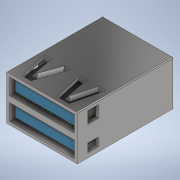
# Autodesk Inventor part: Port 2
Saved by Autodesk Inventor 2020 (Build 240168000, 168)
## iProperties
Created: 2022-11-24
Part Number: Port 2
Material: Generic
Document SubType Name: Modeling
Designer: DELL
Density: 1 g/cm^3
Appearance: Steel - Polished
Author: DELL
Autodesk Inventor part; units mm, degrees
ref_plane "YZ Plane" through (0, 0, 0) normal (1, 0, 0) x (0, 1, 0)
ref_plane "XZ Plane" through (0, 0, 0) normal (0, 1, 0) x (-1, 0, 0)
ref_plane "XY Plane" through (0, 0, 0) normal (0, 0, 1) x (1, 0, 0)
sketch "Sketch1" plane through (0, 0, 0) normal (0, 1, 0) x (-1, 0, 0)
  line L0 (0, 0) -> (0, 32.4)
  line L1 (0, 32.4) -> (-23.897, 32.4)
  line L2 (-23.897, 32.4) -> (-23.897, 0)
  line L3 (-23.897, 0) -> (0, 0)
  dimension "d1" = 32.4
  dimension "d2" = 23.897
  constraints: 8 end point, 3 perpendicular, 1 vertical
  measures "d1" distance of L0.start L0.end
  measures "d2" distance of L0.end L1.end
extrude "Extrusion1" add sketch "Sketch1" along normal blind 15
sketch "Sketch2" plane through (0, 0, 32.4) normal (0, 0, 1) x (1, 0, 0)
  line L0 (23.897, 0) -> (23.897, 15) projected
  line L1 (23.897, 0) -> (0, 0) projected
  line L2 (1, 14) -> (1, 1)
  line L3 (22.897, 14) -> (22.897, 1)
  line L4 (22.897, 14) -> (1, 14)
  line L5 (22.897, 1) -> (1, 1)
  line L6 (1, 14) -> (1, 8.5)
  line L7 (1, 8.5) -> (22.897, 8.5)
  line L8 (1, 1) -> (1, 6.5)
  line L9 (1, 6.5) -> (22.897, 6.5)
  line L10 (1, 14) -> (2, 14)
  line L11 (22.897, 14) -> (21.897, 14)
  line L12 (1, 14) -> (1, 13)
  line L13 (1, 8.5) -> (1, 9.5)
  line L14 (2, 13) -> (2, 9.5)
  line L15 (2, 9.5) -> (21.897, 9.5)
  line L16 (21.897, 9.5) -> (21.897, 13)
  line L17 (21.897, 13) -> (2, 13)
  line L18 (1, 6.5) -> (2, 6.5)
  line L19 (22.897, 6.5) -> (21.897, 6.5)
  line L20 (1, 6.5) -> (1, 5.5)
  line L21 (1, 1) -> (1, 2)
  line L22 (2, 5.5) -> (21.897, 5.5)
  line L23 (21.897, 5.5) -> (21.897, 2)
  line L24 (21.897, 2) -> (2, 2)
  line L25 (2, 2) -> (2, 5.5)
  line L26 (2.5159, 9.5) -> (2.8749, 9.5)
  line L27 (2.8749, 9.5) -> (2.8749, 9.2899)
  line L28 (2.8749, 9.2899) -> (2.5159, 9.2899)
  line L29 (2.5159, 9.2899) -> (2.5159, 9.5)
  line L30 (3.5159, 9.5) -> (3.8749, 9.5)
  line L31 (3.5159, 9.2899) -> (3.5159, 9.5)
  line L32 (3.8749, 9.5) -> (3.8749, 9.2899)
  line L33 (3.8749, 9.2899) -> (3.5159, 9.2899)
  line L34 (4.5159, 9.5) -> (4.8749, 9.5)
  line L35 (4.5159, 9.2899) -> (4.5159, 9.5)
  line L36 (4.8749, 9.5) -> (4.8749, 9.2899)
  line L37 (4.8749, 9.2899) -> (4.5159, 9.2899)
  line L38 (5.5159, 9.5) -> (5.8749, 9.5)
  line L39 (5.5159, 9.2899) -> (5.5159, 9.5)
  line L40 (5.8749, 9.5) -> (5.8749, 9.2899)
  line L41 (5.8749, 9.2899) -> (5.5159, 9.2899)
  line L42 (6.5159, 9.5) -> (6.8749, 9.5)
  line L43 (6.5159, 9.2899) -> (6.5159, 9.5)
  line L44 (6.8749, 9.5) -> (6.8749, 9.2899)
  line L45 (6.8749, 9.2899) -> (6.5159, 9.2899)
  line L46 (7.5159, 9.5) -> (7.8749, 9.5)
  line L47 (7.5159, 9.2899) -> (7.5159, 9.5)
  line L48 (7.8749, 9.5) -> (7.8749, 9.2899)
  line L49 (7.8749, 9.2899) -> (7.5159, 9.2899)
  line L50 (8.5159, 9.5) -> (8.8749, 9.5)
  line L51 (8.5159, 9.2899) -> (8.5159, 9.5)
  line L52 (8.8749, 9.5) -> (8.8749, 9.2899)
  line L53 (8.8749, 9.2899) -> (8.5159, 9.2899)
  line L54 (9.5159, 9.5) -> (9.8749, 9.5)
  line L55 (9.5159, 9.2899) -> (9.5159, 9.5)
  line L56 (9.8749, 9.5) -> (9.8749, 9.2899)
  line L57 (9.8749, 9.2899) -> (9.5159, 9.2899)
  line L58 (10.5159, 9.5) -> (10.8749, 9.5)
  line L59 (10.5159, 9.2899) -> (10.5159, 9.5)
  line L60 (10.8749, 9.5) -> (10.8749, 9.2899)
  line L61 (10.8749, 9.2899) -> (10.5159, 9.2899)
  line L62 (11.5159, 9.5) -> (11.8749, 9.5)
  line L63 (11.5159, 9.2899) -> (11.5159, 9.5)
  line L64 (11.8749, 9.5) -> (11.8749, 9.2899)
  line L65 (11.8749, 9.2899) -> (11.5159, 9.2899)
  line L66 (12.5159, 9.5) -> (12.8749, 9.5)
  line L67 (12.5159, 9.2899) -> (12.5159, 9.5)
  line L68 (12.8749, 9.5) -> (12.8749, 9.2899)
  line L69 (12.8749, 9.2899) -> (12.5159, 9.2899)
  line L70 (13.5159, 9.5) -> (13.8749, 9.5)
  line L71 (13.5159, 9.2899) -> (13.5159, 9.5)
  line L72 (13.8749, 9.5) -> (13.8749, 9.2899)
  line L73 (13.8749, 9.2899) -> (13.5159, 9.2899)
  line L74 (14.5159, 9.5) -> (14.8749, 9.5)
  line L75 (14.5159, 9.2899) -> (14.5159, 9.5)
  line L76 (14.8749, 9.5) -> (14.8749, 9.2899)
  line L77 (14.8749, 9.2899) -> (14.5159, 9.2899)
  line L78 (15.5159, 9.5) -> (15.8749, 9.5)
  line L79 (15.5159, 9.2899) -> (15.5159, 9.5)
  line L80 (15.8749, 9.5) -> (15.8749, 9.2899)
  line L81 (15.8749, 9.2899) -> (15.5159, 9.2899)
  line L82 (16.5159, 9.5) -> (16.8749, 9.5)
  line L83 (16.5159, 9.2899) -> (16.5159, 9.5)
  line L84 (16.8749, 9.5) -> (16.8749, 9.2899)
  line L85 (16.8749, 9.2899) -> (16.5159, 9.2899)
  line L86 (17.5159, 9.5) -> (17.8749, 9.5)
  line L87 (17.5159, 9.2899) -> (17.5159, 9.5)
  line L88 (17.8749, 9.5) -> (17.8749, 9.2899)
  line L89 (17.8749, 9.2899) -> (17.5159, 9.2899)
  line L90 (18.5159, 9.5) -> (18.8749, 9.5)
  line L91 (18.5159, 9.2899) -> (18.5159, 9.5)
  line L92 (18.8749, 9.5) -> (18.8749, 9.2899)
  line L93 (18.8749, 9.2899) -> (18.5159, 9.2899)
  line L94 (19.5159, 9.5) -> (19.8749, 9.5)
  line L95 (19.5159, 9.2899) -> (19.5159, 9.5)
  line L96 (19.8749, 9.5) -> (19.8749, 9.2899)
  line L97 (19.8749, 9.2899) -> (19.5159, 9.2899)
  line L98 (20.5159, 9.5) -> (20.8749, 9.5)
  line L99 (20.5159, 9.2899) -> (20.5159, 9.5)
  line L100 (20.8749, 9.5) -> (20.8749, 9.2899)
  line L101 (20.8749, 9.2899) -> (20.5159, 9.2899)
  line L102 (21.5159, 9.5) -> (21.8749, 9.5)
  line L103 (21.5159, 9.2899) -> (21.5159, 9.5)
  line L104 (21.8749, 9.5) -> (21.8749, 9.2899)
  line L105 (21.8749, 9.2899) -> (21.5159, 9.2899)
  line L106 (2, 2) -> (2.516, 2)
  line L107 (2.516, 2) -> (2.7683, 2)
  line L108 (2.7683, 2) -> (2.7683, 1.8627)
  line L109 (2.7683, 1.8627) -> (2.516, 1.8627)
  line L110 (2.516, 1.8627) -> (2.516, 2)
  line L111 (22.797, 2) -> (2.9, 2)
  line L112 (3.6683, 2) -> (3.6683, 1.8627)
  line L113 (3.416, 2) -> (3.6683, 2)
  line L114 (3.416, 1.8627) -> (3.416, 2)
  line L115 (3.6683, 1.8627) -> (3.416, 1.8627)
  line L116 (23.697, 2) -> (3.8, 2)
  line L117 (4.5683, 2) -> (4.5683, 1.8627)
  line L118 (4.316, 2) -> (4.5683, 2)
  line L119 (4.316, 1.8627) -> (4.316, 2)
  line L120 (4.5683, 1.8627) -> (4.316, 1.8627)
  line L121 (24.597, 2) -> (4.7, 2)
  line L122 (5.4683, 2) -> (5.4683, 1.8627)
  line L123 (5.216, 2) -> (5.4683, 2)
  line L124 (5.216, 1.8627) -> (5.216, 2)
  line L125 (5.4683, 1.8627) -> (5.216, 1.8627)
  line L126 (25.497, 2) -> (5.6, 2)
  line L127 (6.3683, 2) -> (6.3683, 1.8627)
  line L128 (6.116, 2) -> (6.3683, 2)
  line L129 (6.116, 1.8627) -> (6.116, 2)
  line L130 (6.3683, 1.8627) -> (6.116, 1.8627)
  line L131 (26.397, 2) -> (6.5, 2)
  line L132 (7.2683, 2) -> (7.2683, 1.8627)
  line L133 (7.016, 2) -> (7.2683, 2)
  line L134 (7.016, 1.8627) -> (7.016, 2)
  line L135 (7.2683, 1.8627) -> (7.016, 1.8627)
  line L136 (27.297, 2) -> (7.4, 2)
  line L137 (8.1683, 2) -> (8.1683, 1.8627)
  line L138 (7.916, 2) -> (8.1683, 2)
  line L139 (7.916, 1.8627) -> (7.916, 2)
  line L140 (8.1683, 1.8627) -> (7.916, 1.8627)
  line L141 (28.197, 2) -> (8.3, 2)
  line L142 (9.0683, 2) -> (9.0683, 1.8627)
  line L143 (8.816, 2) -> (9.0683, 2)
  line L144 (8.816, 1.8627) -> (8.816, 2)
  line L145 (9.0683, 1.8627) -> (8.816, 1.8627)
  line L146 (29.097, 2) -> (9.2, 2)
  line L147 (9.9683, 2) -> (9.9683, 1.8627)
  line L148 (9.716, 2) -> (9.9683, 2)
  line L149 (9.716, 1.8627) -> (9.716, 2)
  line L150 (9.9683, 1.8627) -> (9.716, 1.8627)
  line L151 (29.997, 2) -> (10.1, 2)
  line L152 (10.8683, 2) -> (10.8683, 1.8627)
  line L153 (10.616, 2) -> (10.8683, 2)
  line L154 (10.616, 1.8627) -> (10.616, 2)
  line L155 (10.8683, 1.8627) -> (10.616, 1.8627)
  line L156 (30.897, 2) -> (11, 2)
  line L157 (11.7683, 2) -> (11.7683, 1.8627)
  line L158 (11.516, 2) -> (11.7683, 2)
  line L159 (11.516, 1.8627) -> (11.516, 2)
  line L160 (11.7683, 1.8627) -> (11.516, 1.8627)
  line L161 (31.797, 2) -> (11.9, 2)
  line L162 (12.6683, 2) -> (12.6683, 1.8627)
  line L163 (12.416, 2) -> (12.6683, 2)
  line L164 (12.416, 1.8627) -> (12.416, 2)
  line L165 (12.6683, 1.8627) -> (12.416, 1.8627)
  line L166 (32.697, 2) -> (12.8, 2)
  line L167 (13.5683, 2) -> (13.5683, 1.8627)
  line L168 (13.316, 2) -> (13.5683, 2)
  line L169 (13.316, 1.8627) -> (13.316, 2)
  line L170 (13.5683, 1.8627) -> (13.316, 1.8627)
  line L171 (33.597, 2) -> (13.7, 2)
  line L172 (14.4683, 2) -> (14.4683, 1.8627)
  line L173 (14.216, 2) -> (14.4683, 2)
  line L174 (14.216, 1.8627) -> (14.216, 2)
  line L175 (14.4683, 1.8627) -> (14.216, 1.8627)
  line L176 (34.497, 2) -> (14.6, 2)
  line L177 (15.3683, 2) -> (15.3683, 1.8627)
  line L178 (15.116, 2) -> (15.3683, 2)
  line L179 (15.116, 1.8627) -> (15.116, 2)
  line L180 (15.3683, 1.8627) -> (15.116, 1.8627)
  line L181 (35.397, 2) -> (15.5, 2)
  line L182 (16.2683, 2) -> (16.2683, 1.8627)
  line L183 (16.016, 2) -> (16.2683, 2)
  line L184 (16.016, 1.8627) -> (16.016, 2)
  line L185 (16.2683, 1.8627) -> (16.016, 1.8627)
  line L186 (36.297, 2) -> (16.4, 2)
  line L187 (17.1683, 2) -> (17.1683, 1.8627)
  line L188 (16.916, 2) -> (17.1683, 2)
  line L189 (16.916, 1.8627) -> (16.916, 2)
  line L190 (17.1683, 1.8627) -> (16.916, 1.8627)
  line L191 (37.197, 2) -> (17.3, 2)
  line L192 (18.0683, 2) -> (18.0683, 1.8627)
  line L193 (17.816, 2) -> (18.0683, 2)
  line L194 (17.816, 1.8627) -> (17.816, 2)
  line L195 (18.0683, 1.8627) -> (17.816, 1.8627)
  line L196 (38.097, 2) -> (18.2, 2)
  line L197 (18.9683, 2) -> (18.9683, 1.8627)
  line L198 (18.716, 2) -> (18.9683, 2)
  line L199 (18.716, 1.8627) -> (18.716, 2)
  line L200 (18.9683, 1.8627) -> (18.716, 1.8627)
  line L201 (38.997, 2) -> (19.1, 2)
  line L202 (19.8683, 2) -> (19.8683, 1.8627)
  line L203 (19.616, 2) -> (19.8683, 2)
  line L204 (19.616, 1.8627) -> (19.616, 2)
  line L205 (19.8683, 1.8627) -> (19.616, 1.8627)
  line L206 (39.897, 2) -> (20, 2)
  line L207 (20.7683, 2) -> (20.7683, 1.8627)
  line L208 (20.516, 2) -> (20.7683, 2)
  line L209 (20.516, 1.8627) -> (20.516, 2)
  line L210 (20.7683, 1.8627) -> (20.516, 1.8627)
  line L211 (40.797, 2) -> (20.9, 2)
  line L212 (21.6683, 2) -> (21.6683, 1.8627)
  line L213 (21.416, 2) -> (21.6683, 2)
  line L214 (21.416, 1.8627) -> (21.416, 2)
  line L215 (21.6683, 1.8627) -> (21.416, 1.8627)
  point P0 (0, 15)
  dimension "d9" = 5.5
  dimension "d10" = 5.5
  dimension "d11" = 1
  dimension "d13" = 1
  dimension "d14" = 1
  dimension "d15" = 1
  dimension "d17" = 1
  dimension "d18" = 1
  dimension "d21" = 1
  dimension "d26" = 0.516
  dimension "d29" = 0.9
  constraints: 424 end point, 202 horizontal alignment, 100 collinear, 84 parallel, 33 point on line, 4 perpendicular, 3 horizontal, 1 vertical, 8 other
  measures "d9" distance of L2.start L6.end
  measures "d10" distance of L2.end L8.end
  measures "d11" distance of L2.start L10.end
  measures "d13" distance of L2.start L12.end
  measures "d14" distance of L6.end L13.end
  measures "d15" distance of L8.end L18.end
  measures "d17" distance of L8.end L20.end
  measures "d18" distance of L2.end L21.end
  measures "d21" distance of L26.start L30.start
  measures "d26" distance of L25.start L106.end
  measures "d29" distance of L23.end L111.start
extrude "Extrusion2" cut sketch "Sketch2" against normal blind 30 contours L4 L3 L7 L2
extrude "Extrusion3" cut sketch "Sketch2" against normal blind 30 contours L9 L3 L5 L2
extrude "Extrusion4" cut sketch "Sketch2" along normal blind 3 contours L17 L16 L15 L14
extrude "Extrusion5" cut sketch "Sketch2" against normal blind 1 contours L24 L25 L22 L23 | L17 L16 L15 L14
extrude "Extrusion6" cut sketch "Sketch2" against normal blind 1.2 contours L15 L27 L28 L29 | L15 L32 L33 L31 | L15 L36 L37 L35 | L15 L40 L41 L39 | L15 L44 L45 L43 | L15 L48 L49 L47 | L15 L52 L53 L51 | L15 L56 L57 L55 | L15 L60 L61 L59 | L72 L73 L71 L15 | L15 L64 L65 L63 | L68 L69 L67 L15
extrude "Extrusion7" cut sketch "Sketch2" against normal blind 1.2 contours L212 L215 L214 L24 | L24 L108 L109 L110 | L207 L210 L209 L24 | L24 L112 L115 L114 | L202 L205 L204 L24 | L24 L117 L120 L119 | L197 L200 L199 L24 | L24 L122 L125 L124 | L192 L195 L194 L24 | L24 L127 L130 L129 | L187 L190 L189 L24 | L24 L132 L135 L134 | L182 L185 L184 L24 | L24 L137 L140 L139 | L177 L180 L179 L24 | L24 L142 L145 L144 | L172 L175 L174 L24 | L24 L147 L150 L149 | L167 L170 L169 L24 | L24 L152 L155 L154 | L162 L165 L164 L24 | L24 L157 L160 L159 | L104 L105 L103 L15 | L100 L101 L99 L15 | L96 L97 L95 L15 | L92 L93 L91 L15 | L88 L89 L87 L15 | L84 L85 L83 L15 | L80 L81 L79 L15 | L76 L77 L75 L15
sketch "Sketch3" plane through (0, 15, 0) normal (0, 1, 0) x (1, 0, 0)
  line L0 (3.884, -30.9795) -> (6.8749, -30.9795)
  line L1 (6.8749, -30.9795) -> (9.9683, -21.9963)
  line L2 (8.1683, -31.2) -> (8.1683, -2.4) projected
  line L3 (5.8749, -31.2) -> (5.8749, -2.4) projected
  line L4 (3.884, -30.9795) -> (1.8307, -21.9963)
  line L5 (1.8307, -21.9963) -> (3.3422, -21.9963)
  line L6 (4.5159, -31.2) -> (4.5159, -2.4) projected
  line L7 (3.3422, -21.9963) -> (4.6255, -28.584)
  line L8 (4.6255, -28.584) -> (6.4221, -28.584)
  line L9 (6.4221, -28.584) -> (8.816, -21.9963)
  line L10 (8.816, -31.2) -> (8.816, -2.4) projected
  line L11 (9.9683, -21.9963) -> (8.816, -21.9963)
  line L12 (15.8749, -31.2) -> (15.8749, -2.4) projected
  line L13 (15.8749, -31.2) -> (19.8964, -31.2)
  line L14 (19.8964, -31.2) -> (22.1129, -22.0866)
  line L15 (22.1129, -22.0866) -> (20.5159, -22.0866)
  line L16 (20.5159, -31.2) -> (20.5159, -2.4) projected
  line L17 (15.8749, -31.2) -> (13.7918, -22.0866)
  line L18 (13.7918, -22.0866) -> (15.4761, -22.0866)
  line L19 (15.4761, -22.0866) -> (16.916, -29.7704)
  line L20 (16.916, -29.7704) -> (18.4705, -29.7704)
  line L21 (16.916, -31.2) -> (16.916, -2.4) projected
  line L22 (18.4705, -29.7704) -> (20.5159, -22.0866)
  point P0 (0, 0)
  constraints: 32 end point, 5 point on line, 3 horizontal, 3 perpendicular, 1 parallel
extrude "Extrusion8" cut sketch "Sketch3" against normal blind 1.2
sketch "Sketch4" plane through (0, 0, 0) normal (-1, 0, 0) x (0, 0, 1)
  line L0 (21.7231, 12.7724) -> (21.7231, 9.7553)
  line L1 (21.7231, 9.7553) -> (25.3436, 9.7553)
  line L2 (31.2, 9.5) -> (2.4, 9.5) projected
  line L3 (25.3436, 9.7553) -> (25.3436, 12.7724)
  line L4 (25.3436, 12.7724) -> (21.7231, 12.7724)
  line L5 (21.7231, 4.0731) -> (21.7231, 1.5588)
  line L6 (21.7231, 1.5588) -> (25.3436, 1.5588)
  line L7 (31.2, 1.8627) -> (2.4, 1.8627) projected
  line L8 (25.3436, 1.5588) -> (25.3436, 4.7771)
  line L9 (25.3436, 4.7771) -> (21.7231, 4.7771)
  line L10 (21.7231, 4.7771) -> (21.7231, 4.0731)
  point P0 (0, 0)
  constraints: 18 end point, 5 perpendicular, 2 parallel, 2 vertical, 1 point on line
extrude "Extrusion9" cut sketch "Sketch4" against normal blind 1.2
sketch "Sketch5" plane through (23.897, 0, 32.4) normal (1, 0, 0) x (0, 0, -1)
  line L0 (3.4674, 12.175) -> (3.4674, 13.0128)
  line L1 (3.4674, 13.0128) -> (7.1098, 13.0128)
  line L2 (7.1098, 13.0128) -> (7.1098, 9.8201)
  line L3 (7.1098, 9.8201) -> (3.4674, 9.8201)
  line L4 (3.4674, 12.175) -> (3.4674, 9.8201)
  line L5 (3.4674, 4.3637) -> (3.4674, 1.5588)
  line L6 (10.6769, 1.5588) -> (7.0564, 1.5588) projected
  line L7 (3.4674, 1.5588) -> (7.0564, 1.5588)
  line L8 (7.0564, 1.5588) -> (7.0564, 4.3637)
  line L9 (7.0564, 1.5588) -> (7.0564, 4.7771) projected
  line L10 (3.4674, 4.3637) -> (7.0564, 4.3637)
  point P0 (32.4, 0)
  constraints: 18 end point, 4 perpendicular, 3 vertical, 1 point on line
extrude "Extrusion10" cut sketch "Sketch5" against normal blind 1.2
chamfer "Chamfer1" distance 0.9 angle 45 1 edges at (16.1961, 15, 25.9285)
chamfer "Chamfer2" distance 0.9 angle 45 9 edges at (18.1511, 15, 29.7704) (19.4932, 15, 25.9285) (14.634, 15, 22.0866) (21.3144, 15, 22.0866) (2.5864, 15, 21.9963) (3.9838, 15, 25.2902) (5.5238, 15, 28.584) (7.619, 15, 25.2902) (9.3921, 15, 21.9963)
chamfer "Chamfer3" distance 0.2 angle 45 1 edges at (11.9485, 13, 31.4)
chamfer "Chamfer4" distance 0.2 angle 45 3 edges at (11.9485, 5.5, 31.4) (11.9485, 2, 31.4) (11.9485, 9.5, 31.4)
chamfer "Chamfer5" distance 0.8 angle 45 1 edges at (23.897, 13.0128, 27.1114)
chamfer "Chamfer6" distance 0.8 angle 45 2 edges at (0, 12.7724, 23.5334) (0, 4.7771, 23.5334)
fillet "Fillet1" radius 0.3 1 edges at (23.897, 15, 16.2)
fillet "Fillet2" radius 0.3 1 edges at (0, 15, 16.2)
fillet "Fillet3" radius 0.3 5 edges at (0.0879, 14.9121, 0) (0, 7.35, 0) (23.8091, 14.9121, 0) (23.897, 7.35, 0) (11.9485, 15, 0)
body "Solid1"
